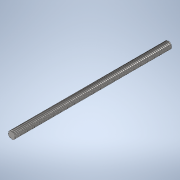
# Autodesk Inventor part: Vitme T8 dai 180mm
Saved by Autodesk Inventor 2020 (Build 240168000, 168)
## iProperties
Created: 2021-05-28
Part Number: Vitme T8 dai 180mm
Material: Generic
Document SubType Name: Modeling
Designer: admin
Density: 1 g/cm^3
Appearance: Galvanized
Author: admin
Autodesk Inventor part; units mm, degrees
ref_plane "YZ Plane" through (0, 0, 0) normal (1, 0, 0) x (0, 1, 0)
ref_plane "XZ Plane" through (0, 0, 0) normal (0, 1, 0) x (-1, 0, 0)
ref_plane "XY Plane" through (0, 0, 0) normal (0, 0, 1) x (1, 0, 0)
sketch "Sketch1" plane through (0, 0, 0) normal (0, 0, 1) x (1, 0, 0)
  circle A0 centre (0, 0) radius 4
  dimension "d0" = 8
  constraints: 1 centre point, 1 coincident
  measures "d0" diameter of A0
extrude "Extrusion1" add sketch "Sketch1" along normal blind 180
sketch "Sketch2" plane through (0, 0, 0) normal (0, 1, 0) x (-1, 0, 0)
  line L0 (4, 0) -> (-4, 0) projected
  circle A0 centre (3.8, 0) radius 0.5
  line L1 (0, -36.6) -> (0, 216.1) projected
  point P0 (0, 0)
  dimension "d3" = 1
  dimension "d4" = 3.8
  constraints: 1 centre point, 1 point on line
  measures "d3" diameter of A0
  measures "d4" distance from line of L1 A0.centre
coil "Coil1" sketch "Sketch2" operation cut axis through (0, 0, -10) along (0, 0, 1) pitch 8 turns 22.5 hand right
pattern_circular "Circular Pattern1" count 4 over 360 about axis through (0, 0, -10) along (0, 0, 1) of "Coil1"
body "Solid1"
